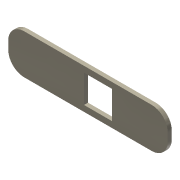
# Autodesk Inventor part: tongue
Saved by Autodesk Inventor 2022 Beta2 (Build 260130000, 130) ContinuousBuild 0
## iProperties
Shininess: 64.0
Length Units: 11272
Angle Units: 11279
Time Units: 11290
Mass Units: 11286
Length Display Precision: 3
Angle Display Precision: 2
Created: 2002-01-23
Part Number: tongue
Vendor: ABC Corp.
Document SubType Name: Modeling
Designer: Administrator
Density: 1 g/cm^3
Material: Generic
Appearance: Light Beige
Density: 0.0
Volumn: 0.0
Area: 0.0
PropertySet Name: Model Information
Control State: 0
Master: False
Checked Out: False
Author: Administrator
Autodesk Inventor part; units mm, degrees
ref_plane "YZ Plane" through (0, 0, 0) normal (1, 0, 0) x (0, 1, 0)
ref_plane "XZ Plane" through (0, 0, 0) normal (0, 1, 0) x (-1, 0, 0)
ref_plane "XY Plane" through (0, 0, 0) normal (0, 0, 1) x (1, 0, 0)
sketch "Sketch1" plane through (0, 0, 0) normal (0, 0, 1) x (1, 0, 0)
  line L0 (-23.2848, 6.1511) -> (27.5152, 6.1511)
  line L1 (27.5152, 6.1511) -> (27.5152, -6.5489)
  line L2 (27.5152, -6.5489) -> (-23.2848, -6.5489)
  line L3 (-23.2848, -6.5489) -> (-23.2848, 6.1511)
  dimension "d0" = 50.8
  dimension "d1" = 12.7
  constraints: 8 end point, 2 parallel, 1 horizontal, 1 perpendicular
  measures "d0" distance of L1.end L2.end
  measures "d1" distance of L2.end L0.start
extrude "Extrusion1" add sketch "Sketch1" along normal blind 1.27
fillet "Fillet1" radius 5.08 4 edges at (-23.2848, 6.1511, 0.635) (27.5152, 6.1511, 0.635) (27.5152, -6.5489, 0.635) (-23.2848, -6.5489, 0.635)
sketch "Sketch2" plane through (0, 0, 1.27) normal (0, 0, 1) x (1, 0, 0)
  line L0 (0.8452, 4.2461) -> (9.7352, 4.2461)
  line L1 (9.7352, 4.2461) -> (9.7352, -4.6439)
  line L2 (9.7352, -4.6439) -> (0.8452, -4.6439)
  line L3 (0.8452, -4.6439) -> (0.8452, 4.2461)
  point P0 (22.4352, -6.5489)
  point P1 (27.5152, -1.4689)
  dimension "d5" = 8.89
  dimension "d6" = 17.78
  dimension "d7" = 1.905
  dimension "d8" = 8.89
  constraints: 8 end point, 2 parallel, 1 horizontal, 1 perpendicular
  measures "d5" distance of L1.end L2.end
  measures "d6" horizontal distance of point (27.515, -1.469) L1.end
  measures "d7" vertical distance of L1.end point (22.435, -6.549)
  measures "d8" distance of L0.end L1.end
extrude "Extrusion2" cut sketch "Sketch2" against normal through all
body "Solid1"
